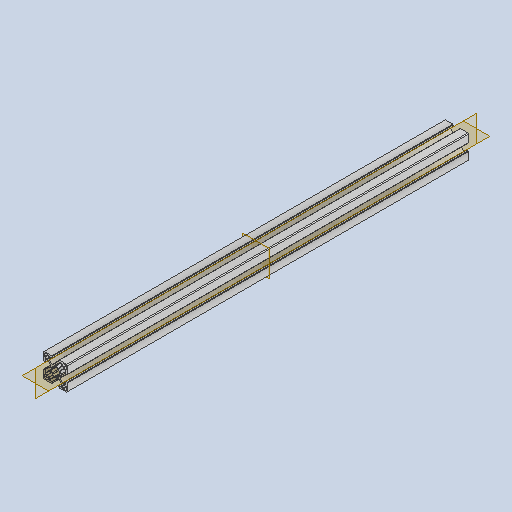
# Autodesk Inventor part: Perfil 30×30 4 rasgos ligeiro_002
Saved by Autodesk Inventor 2026 (Build 300175000, 175)
## iProperties
Created: 2025-04-06
Part Number: Perfil 30×30 4 rasgos ligeiro_002
Material: Aluminum 6061
Document SubType Name: Modeling
Designer: Tony Dias
Density: 2.7 g/cm^3
Appearance: Aluminum - Polished
Author: Tony Dias
Autodesk Inventor part; units mm, degrees
sketch "Sketch1" plane through (0, 0, 0) normal (0, 0, 1) x (1, 0, 0)
  circle A0 centre (0, 0) radius 5 construction
  circle A1 centre (0, 0) radius 5.5 construction
  line L0 (-15, 15) -> (0, 0) construction
  line L1 (-13.75, 13.75) -> (-9.25, 13.75)
  line L2 (-9.25, 13.75) -> (-9.25, 9.25)
  line L3 (-9.25, 9.25) -> (-13.75, 9.25)
  line L4 (-13.75, 9.25) -> (-13.75, 13.75)
  line L5 (-13.75, 13.75) -> (-9.25, 9.25) construction
  line L6 (-9.25, 13.75) -> (-13.75, 9.25) construction
  line L7 (-15, 15) -> (-15, 4.1) construction
  line L8 (-15, 4.1) -> (-12.8, 4.1) construction
  line L9 (-12.8, 8) -> (-12.8, 4.1)
  line L10 (-12.8, 8) -> (-9.5556, 8)
  circle A2 centre (0, 0) radius 6.75 construction
  line L11 (-0.625, 5) -> (0.625, 5) construction
  line L12 (0.625, 5) -> (0.625, 5.4644) construction
  line L13 (-0.625, 5) -> (-0.625, 5.4644)
  arc A3 (0.625, 5.4644) -> (-0.625, 5.4644) centre (0, 0) ccw construction
  line L14 (-3.9775, 3.0936) -> (-4.3058, 3.422)
  line L15 (-3.9775, 3.0936) -> (-3.0936, 3.9775)
  line L16 (-3.0936, 3.9775) -> (-3.422, 4.3058)
  line L17 (-5, -0.625) -> (-5.4644, -0.625) construction
  line L18 (-5, -0.625) -> (-5, 0.625) construction
  line L19 (-5, 0.625) -> (-5.4644, 0.625)
  line L20 (-3.0936, -3.9775) -> (-3.422, -4.3058) construction
  line L21 (-3.0936, -3.9775) -> (-3.9775, -3.0936) construction
  line L22 (-3.9775, -3.0936) -> (-4.3058, -3.422) construction
  line L23 (0.625, -5) -> (0.625, -5.4644) construction
  line L24 (0.625, -5) -> (-0.625, -5) construction
  line L25 (-0.625, -5) -> (-0.625, -5.4644) construction
  line L26 (3.9775, -3.0936) -> (4.3058, -3.422) construction
  line L27 (3.9775, -3.0936) -> (3.0936, -3.9775) construction
  line L28 (3.0936, -3.9775) -> (3.422, -4.3058) construction
  line L29 (5, 0.625) -> (5.4644, 0.625) construction
  line L30 (5, 0.625) -> (5, -0.625) construction
  line L31 (5, -0.625) -> (5.4644, -0.625) construction
  line L32 (3.0936, 3.9775) -> (3.422, 4.3058) construction
  line L33 (3.0936, 3.9775) -> (3.9775, 3.0936) construction
  line L34 (3.9775, 3.0936) -> (4.3058, 3.422) construction
  arc A4 (-0.625, 5.4644) -> (-3.422, 4.3058) centre (0, 0) ccw
  arc A5 (3.422, 4.3058) -> (0.625, 5.4644) centre (0, 0) ccw construction
  arc A6 (5.4644, 0.625) -> (4.3058, 3.422) centre (0, 0) ccw construction
  line L35 (-0.625, 5) -> (0, 5)
  arc A7 (-4.3058, 3.422) -> (-5.4644, 0.625) centre (0, 0) ccw
  line L36 (-5, 0.625) -> (-5, 0)
  line L37 (0, 6.75) -> (0, 5) construction
  line L38 (-0.7864, 6.704) -> (0, 6.25)
  line L39 (-6.704, 0.7864) -> (-6.25, 0)
  line L40 (-9.5556, 8) -> (-5.487, 3.9313)
  line L41 (-8, 9.5556) -> (-3.9313, 5.487)
  line L42 (-15, 15) -> (-4.1, 15) construction
  line L43 (-4.1, 15) -> (-4.1, 12.8) construction
  line L44 (-4.1, 12.8) -> (-8, 12.8)
  line L45 (-8, 12.8) -> (-8, 9.5556)
  arc A8 (-0.7864, 6.704) -> (-3.9313, 5.487) centre (0, 0) ccw
  arc A9 (-5.487, 3.9313) -> (-6.704, 0.7864) centre (0, 0) ccw
  line L46 (-6.25, 0) -> (-5, 0)
  line L47 (0, 5) -> (0, 6.25)
  line L48 (-15, 4.1) -> (-14.5, 4.1) construction
  line L49 (-14.5, 4.1) -> (-14.5, 4.6)
  line L50 (-14.5, 4.6) -> (-15, 4.6)
  line L51 (-15, 4.6) -> (-15, 4.1) construction
  line L52 (-14.5, 4.1) -> (-12.8, 4.1)
  line L53 (-15, 4.6) -> (-15, 15)
  line L54 (-4.1, 15) -> (-4.6, 15) construction
  line L55 (-4.6, 15) -> (-4.6, 14.5)
  line L56 (-4.6, 14.5) -> (-4.1, 14.5)
  line L57 (-4.1, 14.5) -> (-4.1, 15) construction
  line L58 (-4.1, 14.5) -> (-4.1, 12.8)
  line L59 (-4.6, 15) -> (-15, 15)
  point P0 (-11.5, 11.5)
  point P1 (-11.5, 11.5)
  point P2 (-3.5355, 3.5355)
  point P3 (-3.5355, -3.5355)
  point P4 (0, -5)
  point P5 (3.5355, -3.5355)
  point P6 (5, 0)
  point P7 (3.5355, 3.5355)
  dimension "d0" = 10
  dimension "d1" = 0.5
  dimension "d2" = 15
  dimension "d3" = 15
  dimension "d4" = 4.5
  dimension "d5" = 11.5
  dimension "d6" = 11.5
  dimension "d7" = 4.1
  dimension "d8" = 2.2
  dimension "d9" = 1.25
  dimension "d11" = 1.25
  dimension "d12" = 1.25
  dimension "d16" = 360
  dimension "d20" = 1.25
  dimension "d21" = 60
  dimension "d22" = 1.1
  dimension "d23" = 0.5
  constraints: 120 end point, 21 point on circle, 10 centre point, 9 equal length, 8 horizontal, 7 concentric, 7 parallel, 7 vertical, 6 collinear, 4 perpendicular, 3 midpoint, 2 coincident, 1 horizontal alignment, 1 point on line, 1 tangent, 1 vertical alignment, 67 other
  measures "d0" diameter of A0
  measures "d1" radial gap between concentric circles of A0 A1
  measures "d2" horizontal distance of point (0, 0) L0.start
  measures "d3" horizontal distance of point (0, 0) L0.start
  measures "d4" distance of L2.end L3.end
  measures "d5" horizontal distance of point (0, 0) point (-11.5, 11.5)
  measures "d6" horizontal distance of point (0, 0) point (-11.5, 11.5)
  measures "d7" vertical distance of point (0, 0) L7.end
  measures "d8" distance of L7.end L8.end
  measures "d9" distance between parallel lines of L3 L10
  measures "d11" radial gap between concentric circles of A1 A2
  measures "d12" distance of L11.start L11.end
  measures "d20" distance of L35.end L38.end
  measures "d21" angle of L37 L38
  measures "d22" distance between parallel lines of L0 L40
  measures "d23" distance of L49.end L50.end
extrude "Extrusion1" add sketch "Sketch1" along normal mid plane 500
fillet "Fillet1" radius 1 2 edges at (-15, 15, 0) (-13.75, 13.75, 0)
fillet "Fillet2" radius 0.5 9 edges at (-8, 9.5556, 0) (-13.75, 9.25, 0) (-3.9313, 5.487, 0) (-5.487, 3.9313, 0) (-9.25, 9.25, 0) (-9.25, 13.75, 0) (-9.5556, 8, 0) (-12.8, 8, 0) (-8, 12.8, 0)
mirror "Mirror1" about plane through (0, 0, 0) normal (1, 0, 0) of "Extrusion1", "Fillet1", "Fillet2"
mirror "Mirror2" about plane through (0, 0, 0) normal (0, 1, 0) of "Extrusion1", "Fillet1", "Fillet2", "Mirror1"
equation "\"d3\" = d2"
equation "\"d6\" = d5"
equation "\"d12\" = d9"
equation "\"d20\" = d11"
equation "\"d23\" = d1"
body "Solid1"
